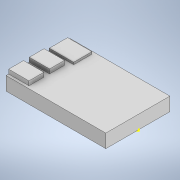
# Autodesk Inventor part: RaspPi_Model
Saved by Autodesk Inventor 2021 (Build 250183000, 183)
## iProperties
Created: 2020-07-08
Part Number: RaspPi_Model
Material: Generic
Document SubType Name: Modeling
Designer: ameli
Density: 1 g/cm^3
Appearance: Default
Author: ameli
Autodesk Inventor part; units mm, degrees
ref_plane "YZ Plane" through (0, 0, 0) normal (1, 0, 0) x (0, 1, 0)
ref_plane "XZ Plane" through (0, 0, 0) normal (0, 1, 0) x (-1, 0, 0)
ref_plane "XY Plane" through (0, 0, 0) normal (0, 0, 1) x (1, 0, 0)
sketch "Sketch1" plane through (0, 0, 0) normal (0, 1, 0) x (-1, 0, 0)
  line L0 (43.575, 28.025) -> (-43.575, 28.025)
  line L1 (-43.575, 28.025) -> (-43.575, -27.975)
  line L2 (-43.575, -27.975) -> (43.575, -27.975)
  line L3 (43.575, -27.975) -> (43.575, 28.025)
  point P0 (0, 0)
  dimension "d0" = 87.15
  dimension "d1" = 56
  dimension "d2" = 27.975
  dimension "d3" = 43.575
  constraints: 8 end point, 2 parallel, 1 horizontal, 1 perpendicular
  measures "d0" distance of L1.end L2.end
  measures "d1" distance of L0.end L1.end
  measures "d2" distance from line of point (0, 0) L2
  measures "d3" distance from line of point (0, 0) L1
extrude "Extrusion1" add sketch "Sketch1" along normal blind 11.8
sketch "Sketch4" plane through (0, 11.8, 0) normal (0, 1, 0) x (1, 0, 0)
  line L0 (-43.575, 25.725) -> (-22.275, 25.725)
  line L1 (-22.275, 25.725) -> (-22.275, 9.725)
  line L2 (-22.275, 9.725) -> (-43.575, 9.725)
  line L3 (-43.575, 9.725) -> (-43.575, 25.725)
  line L4 (-43.575, 5.225) -> (-25.825, 5.225)
  line L5 (-25.825, 5.225) -> (-25.825, -7.775)
  line L6 (-25.825, -7.775) -> (-43.575, -7.775)
  line L7 (-43.575, -7.775) -> (-43.575, 5.225)
  line L8 (-43.575, -12.775) -> (-25.825, -12.775)
  line L9 (-25.825, -12.775) -> (-25.825, -25.775)
  line L10 (-25.825, -25.775) -> (-43.575, -25.775)
  line L11 (-43.575, -25.775) -> (-43.575, -12.775)
  line L12 (43.575, 27.975) -> (-43.575, 27.975) projected
  line L13 (-43.575, 27.975) -> (-43.575, -28.025) projected
  point P0 (0, 0)
  dimension "d7" = 16
  dimension "d8" = 21.3
  dimension "d9" = 2.25
  dimension "d10" = 0
  dimension "d11" = 4.5
  dimension "d12" = 17.75
  dimension "d13" = 13
  dimension "d14" = 5
  dimension "d15" = 13
  dimension "d16" = 17.75
  constraints: 24 end point, 6 parallel, 3 horizontal, 3 perpendicular, 2 point on line
  measures "d7" distance of L0.end L1.end
  measures "d8" distance of L0.start L0.end
  measures "d9" distance between parallel lines of L12 L0
  measures "d10" distance between parallel lines of L13 L3
  measures "d11" distance between parallel lines of L4 L2
  measures "d12" distance of L4.start L4.end
  measures "d13" distance of L4.end L5.end
  measures "d14" distance between parallel lines of L8 L6
  measures "d15" distance of L8.end L9.end
  measures "d16" distance of L8.start L8.end
extrude "Extrusion2" add sketch "Sketch4" along normal blind 3.7 contours L4 L5 L6 L7 | L8 L9 L10 L11
sketch "Sketch6" plane through (0, 11.8, 0) normal (0, 1, 0) x (1, 0, 0)
  line L0 (-43.575, 25.725) -> (-22.275, 25.725)
  line L1 (-22.275, 25.725) -> (-22.275, 9.725)
  line L2 (-22.275, 9.725) -> (-43.575, 9.725)
  line L3 (-43.575, 9.725) -> (-43.575, 25.725)
  line L4 (-43.575, 5.225) -> (-25.825, 5.225) projected
  line L5 (-43.575, 27.975) -> (-43.575, 5.225) projected
  point P0 (0, 0)
  dimension "d19" = 16
  dimension "d20" = 21.3
  dimension "d21" = 4.5
  dimension "d22" = 0
  constraints: 8 end point, 2 parallel, 1 horizontal, 1 perpendicular
  measures "d19" distance of L0.end L1.end
  measures "d20" distance of L1.end L2.end
  measures "d21" distance between parallel lines of L2 L4
  measures "d22" distance between parallel lines of L3 L5
extrude "Extrusion3" add sketch "Sketch6" along normal blind 1.8
sketch "Sketch7" plane through (43.575, 0, -27.975) normal (0, 0, -1) x (-1, 0, 0)
  line L0 (49.95, 7.3) -> (57.15, 7.3)
  line L1 (57.15, 7.3) -> (57.15, 1.4)
  line L2 (57.15, 1.4) -> (49.95, 1.4)
  line L3 (49.95, 1.4) -> (49.95, 7.3)
  line L4 (0, 0) -> (87.15, 0) projected
  line L5 (65.85, 11.8) -> (65.85, 13.6) projected
  point P0 (43.575, 0)
  dimension "d25" = 5.9
  dimension "d26" = 1.4
  dimension "d27" = 7.2
  dimension "d28" = 8.7
  constraints: 8 end point, 2 parallel, 1 horizontal, 1 perpendicular
  measures "d25" distance of L0.end L1.end
  measures "d26" distance between parallel lines of L4 L2
  measures "d27" distance of L0.start L0.end
  measures "d28" distance between parallel lines of L1 L5
extrude "Extrusion4" add sketch "Sketch7" along normal blind 3.5
sketch "Sketch8" plane through (43.575, 0, -27.975) normal (0, 0, -1) x (-1, 0, 0)
  line L0 (24.4, 7.4) -> (39.5, 7.4)
  line L1 (39.5, 7.4) -> (39.5, 1.3)
  line L2 (39.5, 1.3) -> (24.4, 1.3)
  line L3 (24.4, 1.3) -> (24.4, 7.4)
  line L4 (49.95, 1.4) -> (49.95, 7.3) projected
  line L5 (0, 0) -> (87.15, 0) projected
  point P0 (43.575, 0)
  dimension "d31" = 10.45
  dimension "d32" = 15.1
  dimension "d33" = 6.1
  dimension "d34" = 1.3
  constraints: 8 end point, 2 parallel, 1 horizontal, 1 perpendicular
  measures "d31" distance between parallel lines of L4 L1
  measures "d32" distance of L0.start L0.end
  measures "d33" distance of L2.end L0.start
  measures "d34" distance between parallel lines of L5 L2
extrude "Extrusion5" add sketch "Sketch8" along normal blind 2.5
sketch "Sketch9" plane through (43.575, 0, -27.975) normal (0, 0, -1) x (-1, 0, 0)
  line L0 (6.6, 4) -> (14.2, 4)
  line L1 (14.2, 4) -> (14.2, 1.3)
  line L2 (14.2, 1.3) -> (6.6, 1.3)
  line L3 (6.6, 1.3) -> (6.6, 4)
  line L4 (0, 0) -> (87.15, 0) projected
  line L5 (24.4, 1.3) -> (24.4, 7.4) projected
  point P0 (43.575, 0)
  dimension "d37" = 7.6
  dimension "d38" = 2.7
  dimension "d39" = 1.3
  dimension "d40" = 10.2
  constraints: 8 end point, 2 parallel, 1 horizontal, 1 perpendicular
  measures "d37" distance of L0.start L0.end
  measures "d38" distance of L0.end L1.end
  measures "d39" distance between parallel lines of L4 L2
  measures "d40" distance between parallel lines of L5 L1
extrude "Extrusion6" add sketch "Sketch9" along normal blind 2.25
sketch "Sketch10" plane through (43.575, 0, 28.025) normal (1, 0, 0) x (0, 0, -1)
  point P0 (28.025, 0)
body "Solid1"
